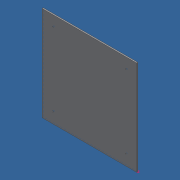
# Autodesk Inventor part: heatbed
Saved by Autodesk Inventor 2021 (Build 250183000, 183)
## iProperties
Created: 2022-08-30
Part Number: heatbed
Material: Generic
Document SubType Name: Modeling
Designer: Nathann
Density: 1 g/cm^3
Appearance: Default
Author: Nathann
Autodesk Inventor part; units mm, degrees
ref_plane "YZ Plane" through (0, 0, 0) normal (1, 0, 0) x (0, 1, 0)
ref_plane "XZ Plane" through (0, 0, 0) normal (0, 1, 0) x (-1, 0, 0)
ref_plane "XY Plane" through (0, 0, 0) normal (0, 0, 1) x (1, 0, 0)
sketch "Sketch1" plane through (0, 0, 0) normal (0, 1, 0) x (-1, 0, 0)
  line L0 (0, 0) -> (310, 0)
  line L1 (310, 0) -> (310, 310)
  line L2 (310, 310) -> (0, 310)
  line L3 (0, 310) -> (0, 0)
  circle A0 centre (35, 35) radius 1.75
  circle A1 centre (275, 35) radius 1.75
  circle A2 centre (35, 275) radius 1.75
  circle A3 centre (275, 275) radius 1.75
  dimension "d0" = 310
  dimension "d1" = 310
  dimension "d2" = 240
  dimension "d3" = 240
  dimension "d4" = 240
  dimension "d5" = 240
  dimension "d6" = 35
  dimension "d7" = 35
  dimension "d8" = 3.5
  dimension "d9" = 3.5
  dimension "d10" = 3.5
  dimension "d11" = 3.5
  constraints: 8 end point, 4 centre point, 2 parallel, 1 horizontal, 1 perpendicular
  measures "d0" distance of L1.end L2.end
  measures "d1" distance of L2.end L0.start
  measures "d2" distance of A0.centre A1.centre
  measures "d3" distance of A0.centre A2.centre
  measures "d4" distance of A1.centre A3.centre
  measures "d5" distance of A2.centre A3.centre
  measures "d6" distance from line of L3 A0.centre
  measures "d7" distance from line of L0 A0.centre
  measures "d8" diameter of A3
  measures "d9" diameter of A1
  measures "d10" diameter of A0
  measures "d11" diameter of A2
extrude "Extrusion1" add sketch "Sketch1" along normal blind 4
sketch "Sketch2" plane through (0, 4, 0) normal (0, 1, 0) x (1, 0, 0)
  line L0 (-298.7801, -142.1723) -> (8.953, -142.1723) construction
  line L1 (8.953, -142.1723) -> (8.953, -252.6087) construction
  line L2 (8.953, -252.6087) -> (-298.7801, -252.6087) construction
  line L3 (-298.7801, -252.6087) -> (-298.7801, -142.1723) construction
  point P0 (0, 0)
  constraints: 2 other
equation "\"d6\" = -0.5 * d2 + 0.5 * d1"
equation "\"d7\" = -0.5 * d2 + 0.5 * d1"
equation "\"d9\" = d8"
body "Solid1"
